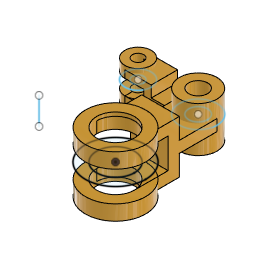
Tutorial5 v2 (Autodesk Fusion 360 design; units mm, degrees)
Autodesk Fusion 360 part; units mm, degrees
sketch "Sketch1" plane through (0, 0, 0) normal (0, 0, 1) x (1, 0, 0)
  circle A0 centre (0, 0) radius 25
  circle A1 centre (0, 0) radius 40
  circle A2 centre (0, 110) radius 12.5
  circle A3 centre (0, 110) radius 25
  circle A4 centre (-80, 110) radius 7.5
  circle A5 centre (-80, 110) radius 17.5
  dimension "d5" = 50
  dimension "d6" = 80
  dimension "d7" = 25
  dimension "d8" = 50
  dimension "d9" = 110
  dimension "d10" = 15
  dimension "d11" = 35
  dimension "d12" = 80
  constraint coincident A0.centre A1.centre
  constraint concentric A0 A1
  constraint concentric A2 A3
  constraint concentric A4 A5
  measures "d5" diameter of A0
  measures "d6" diameter of A1
  measures "d7" diameter of A2
  measures "d8" diameter of A3
  measures "d9" distance of A0.centre A2.centre
  measures "d10" diameter of A4
  measures "d11" diameter of A5
  measures "d12" distance of A2.centre A4.centre
extrude "Extrude1" add sketch "Sketch1" along normal blind 10 from surface at 20 contours A1 makes body 1
extrude "Extrude2" add sketch "Sketch1" against normal blind 10 from surface at -20 separate body contours A1 makes body 2
extrude "Extrude3" add sketch "Sketch1" along normal blind 15 from surface at 10 separate body contours A5 makes body 3
extrude "Extrude4" add sketch "Sketch1" against normal blind 15 from surface at -10 separate body contours A5 makes body 4
extrude "Extrude5" add sketch "Sketch1" along normal mid plane 60 separate body contours A3 makes body 5
extrude "Extrude6" add 1 faces at (34.758, -3.2292, 30) along direction (0, 0, 1) blind 10 on bodies 1 bodies 1
extrude "Extrude7" add 1 faces at (34.758, -3.2292, -30) along direction (0, 0, -1) blind 10 on bodies 2 bodies 2
sketch "Sketch3" plane through (0, 0, 0) normal (1, 0, 0) x (0, 1, 0)
  line L0 (0, 20) -> (45, 20)
  line L1 (45, 20) -> (45, 35)
  line L2 (45, 35) -> (0, 35)
  line L3 (0, 35) -> (0, 20)
  line L4 (0, -20) -> (45, -20)
  line L5 (45, -20) -> (45, -35)
  line L6 (45, -35) -> (0, -35)
  line L7 (0, -35) -> (0, -20)
  line L8 (45, -35) -> (60, -35)
  line L9 (60, -35) -> (60, 35)
  line L10 (60, 35) -> (45, 35)
  line L11 (45, 35) -> (45, -35)
  line L12 (45, -7.5) -> (110, -7.5)
  line L13 (110, -7.5) -> (110, 7.5)
  line L14 (110, 7.5) -> (45, 7.5)
  line L15 (45, 7.5) -> (45, -7.5)
  dimension "d33" = 45
  dimension "d34" = 15
  dimension "d35" = 45
  dimension "d36" = 15
  dimension "d37" = 15
  dimension "d38" = 70
  dimension "d39" = 65
  dimension "d40" = 15
  dimension "d41" = 27.5
  dimension "d42" = 27.5
  constraint horizontal L0
  constraint vertical L1
  constraint horizontal L2
  constraint vertical L3
  constraint horizontal L4
  constraint vertical L5
  constraint horizontal L6
  constraint vertical L7
  constraint horizontal L8
  constraint vertical L9
  constraint horizontal L10
  constraint vertical L11
  constraint horizontal L12
  constraint vertical L13
  constraint horizontal L14
  constraint vertical L15
  constraint coincident L11 L12.start
  measures "d33" distance of L0.start L0.end
  measures "d34" distance of L0.end L1.end
  measures "d35" distance of L4.start L4.end
  measures "d36" distance of L4.end L5.end
  measures "d37" distance of L5.end L8.end
  measures "d38" distance of L8.end L9.end
  measures "d39" distance of L12.start L12.end
  measures "d40" distance of L12.start L14.end
  measures "d41" distance of L10 L14
  measures "d42" distance of L8 L12
extrude "Extrude8" add sketch "Sketch3" along normal mid plane 50 separate body makes body 6
extrude "Extrude9" cut sketch "Sketch1" along normal mid plane 144.06 contours A2 bodies 6
extrude "Extrude10" cut sketch "Sketch1" along normal mid plane 135.33 contours A0 bodies 6
sketch "Sketch4" plane through (0, 0, 0) normal (0, 1, 0) x (1, 0, 0)
  line L0 (-101.7969, -25.8958) -> (-101.7969, 10)
  constraint vertical L0
ref_plane "WorkPlane1" through (-80, 110, 17.5) normal (0, 1, 0) x (0, 0, 1)
sketch "Sketch5" plane through (-80, 110, 17.5) normal (0, 1, 0) x (1, 0, 0)
  line L0 (17.5, 42.5) -> (-17.5, 42.5)
  line L1 (-17.5, 27.5) -> (17.5, 27.5)
  line L2 (17.5, 27.5) -> (17.5, 42.5)
  line L3 (-17.5, 27.5) -> (-17.5, 42.5)
  line L4 (-17.5, -7.5) -> (17.5, -7.5)
  line L5 (-17.5, 7.5) -> (17.5, 7.5)
  line L6 (-17.5, 7.5) -> (-17.5, -7.5)
  line L7 (17.5, 7.5) -> (17.5, -7.5)
  line L8 (105, 47.5) -> (55, 47.5)
  line L9 (55, -12.5) -> (105, -12.5)
  line L10 (55, 47.5) -> (55, -12.5)
  line L11 (105, 47.5) -> (105, -12.5)
  line L12 (0, 7.5) -> (25, 7.5)
  line L13 (25, 7.5) -> (25, -2.5)
  line L14 (25, -2.5) -> (0, -2.5)
  line L15 (0, -2.5) -> (0, 7.5)
  line L16 (0, 27.5) -> (25, 27.5)
  line L17 (25, 27.5) -> (25, 37.5)
  line L18 (25, 37.5) -> (0, 37.5)
  line L19 (0, 37.5) -> (0, 27.5)
  line L20 (25, 37.5) -> (35, 37.5)
  line L21 (35, 37.5) -> (35, -2.5)
  line L22 (35, -2.5) -> (25, -2.5)
  line L23 (25, -2.5) -> (25, 37.5)
  line L24 (25, 22.4841) -> (80, 22.4841)
  line L25 (80, 22.4841) -> (80, 12.4841)
  line L26 (80, 12.4841) -> (25, 12.4841)
  line L27 (25, 12.4841) -> (25, 22.4841)
  dimension "d53" = 25
  dimension "d54" = 10
  dimension "d55" = 25
  dimension "d56" = 10
  dimension "d57" = 10
  dimension "d58" = 55
  dimension "d59" = 10
  constraint horizontal L12
  constraint vertical L13
  constraint horizontal L14
  constraint vertical L15
  constraint midpoint L5 L12.start
  constraint horizontal L16
  constraint vertical L17
  constraint horizontal L18
  constraint vertical L19
  constraint midpoint L1 L16.start
  constraint horizontal L20
  constraint vertical L21
  constraint horizontal L22
  constraint vertical L23
  constraint coincident L14 L21.end
  constraint horizontal L24
  constraint vertical L25
  constraint horizontal L26
  constraint vertical L27
  constraint coincident L23 L24.start
  measures "d53" distance of L12.start L12.end
  measures "d54" distance of L12.start L14.end
  measures "d55" distance of L16.start L16.end
  measures "d56" distance of L16.start L18.end
  measures "d57" distance of L17.end L20.end
  measures "d58" distance of L24.start L24.end
  measures "d59" distance of L24.end L25.end
extrude "Extrude11" add sketch "Sketch5" along normal mid plane 35 separate body contours L2 L16 L17 L18 L23 | L1 L2 L16 L18 L19 | L17 L20 L21 L23 L24 | L21 L23 L24 L26 L27 | L10 L21 L24 L26 | L13 L21 L22 L23 L26 | L10 L24 L25 L26 | L7 L12 L13 L14 L23 | L5 L7 L12 L14 L15 makes body 7
extrude "Extrude12" cut sketch "Sketch1" along normal mid plane 104.95 contours A2 bodies 7
extrude "Extrude13" cut sketch "Sketch1" along normal mid plane 79.018 contours A4 bodies 7
